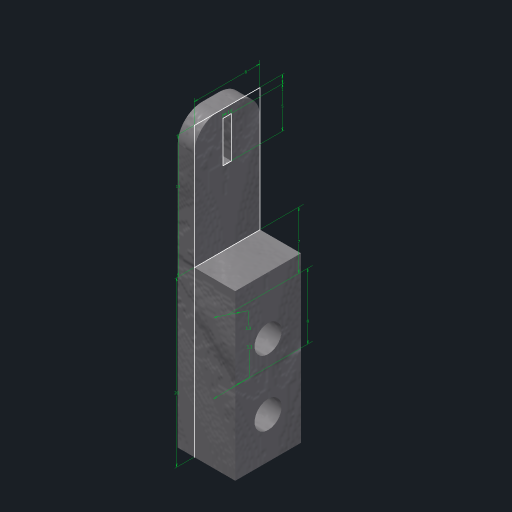
# Autodesk Inventor part: MUESCA_DETECCION_CERO
Saved by Autodesk Inventor 2024.3 (Build 283343000, 343)
## iProperties
Created: 2024-07-13
Part Number: MUESCA_DETECCION_CERO
Material: Steel, Mild, Welded
Document SubType Name: Modeling
Designer: Niler
Density: 7.85 g/cm^3
Appearance: Weld - Steel Mild
Author: Niler
Autodesk Inventor part; units mm, degrees
ref_plane "YZ Plane" through (0, 0, 0) normal (1, 0, 0) x (0, 1, 0)
ref_plane "XZ Plane" through (0, 0, 0) normal (0, 1, 0) x (-1, 0, 0)
ref_plane "XY Plane" through (0, 0, 0) normal (0, 0, 1) x (1, 0, 0)
sketch "Sketch1" plane through (0, 0, 0) normal (1, 0, 0) x (0, 1, 0)
  line L0 (35, 4) -> (0, 4)
  line L1 (0, 4) -> (0, -4)
  line L2 (0, -4) -> (35, -4)
  line L3 (35, -4) -> (35, 4)
  line L4 (34, 0.5) -> (29, 0.5)
  line L5 (29, 0.5) -> (29, -0.5)
  line L6 (29, -0.5) -> (34, -0.5)
  line L7 (34, -0.5) -> (34, 0.5)
  line L8 (20, 4) -> (20, -4)
  circle A0 centre (13, 0) radius 1.65
  circle A1 centre (5, 0) radius 1.65
  point P0 (0, 0)
  point P1 (0, 0)
  point P2 (29, 0)
  point P3 (20, 0)
  dimension "d0" = 8
  dimension "d2" = 1
  dimension "d3" = 1
  dimension "d4" = 5
  dimension "d5" = 20
  dimension "d6" = 15
  dimension "d7" = 3.3
  dimension "d8" = 3.3
  dimension "d9" = 7
  dimension "d10" = 8
  constraints: 18 end point, 4 parallel, 3 horizontal alignment, 3 midpoint, 3 perpendicular, 2 centre point, 2 horizontal, 2 point on line, 1 coincident
  measures "d0" distance of L2.end L0.start
  measures "d2" distance of L6.end L4.start
  measures "d3" distance between parallel lines of L7 L3
  measures "d4" distance of L5.end L6.end
  measures "d5" distance between parallel lines of L1 L8
  measures "d6" distance between parallel lines of L3 L8
  measures "d7" diameter of A0
  measures "d8" diameter of A1
  measures "d9" distance from line of L8 A0.centre
  measures "d10" distance of A1.centre A0.centre
extrude "Extrusion1" add sketch "Sketch1" along normal blind 5 contours L8 L2 L1 L0
extrude "Extrusion2" add sketch "Sketch1" against normal blind 2
fillet "Fillet1" radius 3 2 edges at (-1, 35, 4) (-1, 35, -4)
body "Solid1"
